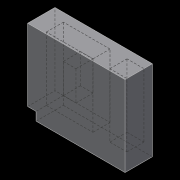
# Autodesk Inventor part: switchback-logo-01
Saved by Autodesk Inventor 2020 (Build 240168000, 168)
## iProperties
Created: 2020-01-09
Part Number: switchback-logo-01
Material: Generic
Document SubType Name: Modeling
Designer: valer
Density: 1 g/cm^3
Appearance: Default
Author: valer
Autodesk Inventor part; units mm, degrees
ref_plane "YZ Plane" through (0, 0, 0) normal (1, 0, 0) x (0, 1, 0)
ref_plane "XZ Plane" through (0, 0, 0) normal (0, 1, 0) x (-1, 0, 0)
ref_plane "XY Plane" through (0, 0, 0) normal (0, 0, 1) x (1, 0, 0)
sketch "TopProfile" plane through (0, 0, 0) normal (0, 0, 1) x (1, 0, 0)
  line L0 (0, 19.6865) -> (0, 0)
  line L1 (9.1702, 14.4367) -> (5.2497, 14.4367)
  line L2 (5.2497, 14.4367) -> (5.2497, 5.2497)
  line L3 (5.2497, 5.2497) -> (9.1702, 5.2497)
  line L4 (9.1702, 5.2497) -> (9.1702, 14.4367)
  line L5 (19.6697, 0) -> (24.9194, 0)
  line L6 (24.9194, 0) -> (24.9194, 19.6865)
  line L7 (24.9194, 19.6865) -> (19.6697, 19.6865)
  line L8 (19.6697, 19.6865) -> (19.6697, 0)
  line L9 (-2.6249, 0) -> (-2.6249, 22.3113)
  line L10 (-2.6249, 22.3113) -> (27.5442, 22.3113)
  line L11 (27.5442, 22.3113) -> (27.5442, -2.6249)
  line L12 (27.5442, -2.6249) -> (0, -2.6249)
  line L13 (0, -2.6249) -> (0, 0)
  line L14 (0, 0) -> (-2.6249, 0)
  line L15 (14.4199, 0) -> (14.4199, 19.6865)
  line L16 (14.4199, 19.6865) -> (0, 19.6865)
  line L17 (0, 0) -> (14.4199, 0)
  line L18 (-2.6249, 0) -> (-2.6249, -2.6249)
  line L19 (-2.6249, -2.6249) -> (0, -2.6249)
  dimension "d3" = 3.9205
  dimension "d4" = 5.2497
  dimension "d8" = 5.2497
  dimension "d12" = 5.2497
  dimension "d13" = 2.6249
  dimension "d14" = 5.2497
  dimension "d15" = 5.2497
  dimension "d16" = 2.6249
  dimension "d17" = 2.6249
  dimension "d18" = 2.6249
  dimension "d19" = 24.9362
  dimension "d20" = 27.5443
  dimension "d21" = 5.2497
  constraints: 40 end point, 7 perpendicular, 3 collinear, 3 parallel, 1 coincident, 1 horizontal, 1 vertical
  measures "d3" distance between parallel lines of L2 L4
  measures "d4" distance between parallel lines of L2 L0
  measures "d8" distance between parallel lines of L6 L8
  measures "d12" distance between parallel lines of L8 L15
  measures "d13" distance between parallel lines of L10 L16
  measures "d14" distance between parallel lines of L15 L4
  measures "d15" distance between parallel lines of L17 L3
  measures "d16" distance between parallel lines of L12 L5
  measures "d17" distance between parallel lines of L11 L6
  measures "d18" distance between parallel lines of L9 L0
  measures "d19" distance of L10.end L12.start
  measures "d20" distance of L12.start L12.end
  measures "d21" distance between parallel lines of L16 L1
extrude "NegativeFeature" add sketch "TopProfile" against normal blind 11.43 contours L14 L9 L10 L11 L12 L13 | L4 L3 L2 L1
extrude "PositiveFeature" add sketch "TopProfile" against normal blind 3.175 contours L16 L15 L17 L0 | L8 L7 L6 L5
body "Solid1"
